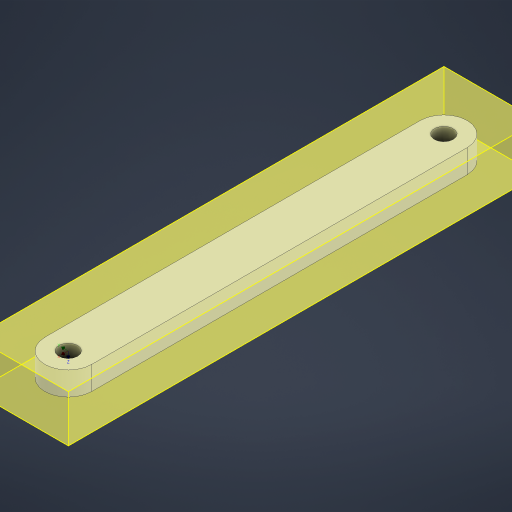
# Autodesk Inventor part: Main Linkage
Saved by Autodesk Inventor 2023 (Build 270158000, 158)
## iProperties
Created: 2022-05-02
Part Number: Main Linkage
Material: Generic
Document SubType Name: Modeling
Designer: FizzyApple12
Density: 1 g/cm^3
Appearance: Default
Author: FizzyApple12
Autodesk Inventor part; units mm, degrees
ref_plane "YZ Plane" through (0, 0, 0) normal (1, 0, 0) x (0, 1, 0)
ref_plane "XZ Plane" through (0, 0, 0) normal (0, 1, 0) x (-1, 0, 0)
ref_plane "XY Plane" through (0, 0, 0) normal (0, 0, 1) x (1, 0, 0)
sketch "Sketch1" plane through (0, 0, 0) normal (0, 1, 0) x (-1, 0, 0)
  circle A0 centre (0, 0) radius 6.35
  circle A1 centre (0, -101.6) radius 6.35
  line L0 (0, 0) -> (0, -109.4726) construction
  line L1 (6.35, -101.6) -> (6.35, 0)
  line L2 (-6.35, -101.6) -> (-6.35, 0)
  dimension "d0" = 101.6
  dimension "d1" = 12.7
  dimension "d2" = 12.7
  constraints: 6 end point, 4 point on circle, 4 tangent, 3 coincident, 2 centre point, 1 point on line, 1 vertical
  measures "d0" distance of point (0, -101.6) point (0, 0)
  measures "d1" diameter of A0
  measures "d2" diameter of A1
extrude "Extrusion1" add sketch "Sketch1" along normal blind 6.35
hole "Hole1" at (0, 0, 0) at (0, 0, -101.6) direction (0, 1, 0) diameter 5.1054 depth 13.6144 clearance for "Flat Head Machine Screw (82)" size "#10" standard "Ansi Unified Screw Threads"
chamfer "Chamfer1" [suppressed]
body "Solid1"
